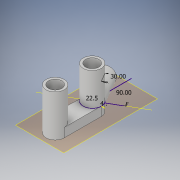
# Autodesk Inventor part: 2 axis end
Saved by Autodesk Inventor 2019 (Build 230136000, 136)
## iProperties
Created: 2018-10-04
Part Number: 2 axis end
Material: Generic
Document SubType Name: Modeling
Designer: HIVE
Density: 1 g/cm^3
Appearance: Default
Author: HIVE
## iProperties of the stored document 2 axis end_3DPrint.ipt
Created: 2018-10-05
Part Number: 2 axis end_3DPrint
Material: Generic
Document SubType Name: Modeling
Designer: Hive
Density: 1 g/cm^3
Appearance: Default
Author: Hive
Autodesk Inventor part; units mm, degrees
ref_plane "YZ Plane" through (0, 0, 0) normal (1, 0, 0) x (0, 1, 0)
ref_plane "XY Plane" through (0, 0, 0) normal (0, 0, 1) x (1, 0, 0)
sketch "Sketch1" plane through (0, 0, 0) normal (0, 1, 0) x (-1, 0, 0)
  circle A0 centre (0, 0) radius 11.25
  circle A1 centre (0, 0) radius 15.25
  line L0 (-15.25, 0) -> (15.25, 0)
  arc A2 (-15.25, 0) -> (15.25, 0) centre (0, 0) ccw
  line L1 (21.35, 0) -> (-21.35, 0) projected
  dimension "d0" = 22.5
  dimension "d1" = 4
  constraints: 4 point on circle, 3 centre point, 2 coincident, 2 end point, 1 horizontal
  measures "d0" diameter of A0
  measures "d1" radial gap between concentric circles of A0 A1
extrude "Extrusion1" add sketch "Sketch1" along normal blind 55 contours L0 A1 A0 | A0 L0 A1
extrude "Extrusion2" add sketch "Sketch1" along normal blind 15.25 contours L0 A0 | A0 L0
pattern_linear "Rectangular Pattern1" count 2 spacing 62.5 along (0, 0, 1) of "Extrusion1", "Extrusion2"
sketch "Sketch2" plane through (0, 0, 0) normal (0, 1, 0) x (-1, 0, 0)
  circle A0 centre (0, 0) radius 11.25 projected
  line L0 (0, 0) -> (20.7638, -35.964)
  line L1 (0, 0) -> (0, -66.0137)
  line L2 (0, 0) -> (-33.2364, -19.1891)
  dimension "d16" = 30
  dimension "d17" = 90
  constraints: 6 end point, 1 vertical
  measures "d16" angle of L1 L0
  measures "d17" angle of L0 L2
pattern_circular "Circular Pattern3" count 2 over 90 about axis through (0, 0, 0) along (-0.8660254, 0, 0.5) of "Extrusion1", "Extrusion2"
sketch "Sketch3" plane through (0, 0, 0) normal (0, 1, 0) x (-1, 0, 0)
  circle A0 centre (0, 62.5) radius 15.25 projected
  line L0 (13.2069, 7.625) -> (-13.2069, -7.625) projected
  arc A1 (13.2069, 7.625) -> (-13.2069, -7.625) centre (0, 0) ccw projected
  circle A2 centre (0, 62.5) radius 15.25 projected
  line L1 (15.25, 62.5) -> (13.2069, 7.625)
  line L2 (-15.25, 62.5) -> (-15.25, 0)
  constraints: 4 end point, 3 point on circle, 1 tangent
ref_plane "Work Plane1" through (0, -15.25, 0) normal (0, 1, 0) x (-1, 0, 0)
extrude "Extrusion3" add sketch "Sketch3" against normal up to surface (15.25 mm away) contours L1 A0 | A0 L1 A1 L2 | A1 L0 picked at (2.685, 66.663)
equation "\"calc\" = 34.75"
body "Solid1"
